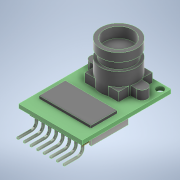
# Autodesk Inventor part: Camera
Saved by Autodesk Inventor 2022 (Build 260153000, 153)
## iProperties
Created: 2022-12-31
Part Number: Camera
Material: Generic
Document SubType Name: Modeling
Designer: karpova
Density: 1 g/cm^3
Appearance: Smooth - Dark Forest Green
Author: karpova
Autodesk Inventor part; units mm, degrees
ref_plane "YZ Plane" through (0, 0, 0) normal (1, 0, 0) x (0, 1, 0)
ref_plane "XZ Plane" through (0, 0, 0) normal (0, 1, 0) x (-1, 0, 0)
ref_plane "XY Plane" through (0, 0, 0) normal (0, 0, 1) x (1, 0, 0)
sketch "Sketch1" plane through (0, 0, 0) normal (0, 1, 0) x (-1, 0, 0)
  line L0 (0, 0) -> (34.25, 0)
  line L1 (34.25, 0) -> (34.25, -24.4)
  line L2 (34.25, -24.4) -> (0, -24.4)
  line L3 (0, -24.4) -> (0, 0)
  dimension "d0" = 24.4
  dimension "d1" = 34.25
  constraints: 8 end point, 2 parallel, 1 horizontal, 1 perpendicular
  measures "d0" distance of L0.end L1.end
  measures "d1" distance of L0.start L0.end
extrude "Extrusion1" add sketch "Sketch1" along normal blind 1.54
sketch "Sketch4" plane through (0, 1.54, 0) normal (0, 1, 0) x (1, 0, 0)
  line L0 (-32.8, 5.675) -> (-19.75, 5.675)
  line L1 (-19.75, 5.675) -> (-19.75, 18.725)
  line L2 (-19.75, 18.725) -> (-32.8, 18.725)
  line L3 (-32.8, 18.725) -> (-32.8, 5.675)
  circle A0 centre (-32.12, 2.2) radius 1.5 projected
  line L4 (-34.25, 24.4) -> (-34.25, 0) construction
  line L5 (-34.25, 12.2) -> (0, 12.2) construction
  line L6 (0, 0) -> (0, 24.4) construction
  line L7 (-26.275, 18.725) -> (-26.275, 5.675) construction
  line L8 (-28.325, 18.725) -> (-24.225, 18.725)
  line L9 (-24.225, 18.725) -> (-24.225, 21.2)
  line L10 (-26.275, 23.25) -> (-26.275, 23.25)
  line L11 (-28.325, 21.2) -> (-28.325, 18.725)
  line L12 (-24.225, 5.675) -> (-24.225, 3.2)
  line L13 (-26.275, 1.15) -> (-26.275, 1.15)
  line L14 (-28.325, 3.2) -> (-28.325, 5.675)
  arc A1 (-26.275, 23.25) -> (-28.325, 21.2) centre (-26.275, 21.2) ccw
  arc A2 (-24.225, 21.2) -> (-26.275, 23.25) centre (-26.275, 21.2) ccw
  arc A3 (-28.325, 3.2) -> (-26.275, 1.15) centre (-26.275, 3.2) ccw
  arc A4 (-26.275, 1.15) -> (-24.225, 3.2) centre (-26.275, 3.2) ccw
  point P0 (-24.225, 23.25)
  point P1 (-28.325, 23.25)
  point P2 (-24.225, 1.15)
  point P3 (-28.325, 1.15)
  point P4 (-26.275, 1.15)
  dimension "d43" = 13.05
  dimension "d44" = 14.5
  dimension "d56" = 4.1
  dimension "d57" = 22.1
  dimension "d58" = 2.05
  constraints: 26 end point, 9 point on line, 8 point on circle, 8 tangent, 4 centre point, 4 midpoint, 4 symmetric about line, 3 equal radius, 3 parallel, 3 perpendicular, 2 horizontal, 1 vertical, 2 other
  measures "d43" distance between parallel lines of L2 L0
  measures "d44" distance between parallel lines of L4 L1
  measures "d56" distance between parallel lines of L9 L11
  measures "d57" distance between parallel lines of L10 L13
  measures "d58" radius of A1
extrude "Extrusion2" add sketch "Sketch4" along normal blind 3.46 contours L3 L2 L1 L0 | L0 L12 A4 A3 L14 | L11 A1 A2 L9 L2
sketch "Sketch8" plane through (0, 1.54, 0) normal (0, 1, 0) x (1, 0, 0)
  line L0 (0, 24.4) -> (-34.25, 24.4) projected
  line L1 (0, 0) -> (0, 24.4) projected
  line L2 (-34.25, 0) -> (0, 0) projected
  line L3 (-34.25, 24.4) -> (-34.25, 0) projected
  line L4 (-32.8, 5.675) -> (-32.8, 18.725) construction
  line L5 (-32.8, 12.2) -> (-26.275, 12.2) construction
  line L6 (-26.275, 12.2) -> (-26.275, 18.725) construction
  line L7 (-32.8, 18.725) -> (-19.75, 18.725) construction
  circle A0 centre (-26.275, 12.2) radius 7
  dimension "d45" = 14
  constraints: 4 end point, 2 midpoint, 1 centre point, 1 coincident, 1 horizontal, 1 vertical
  measures "d45" diameter of A0
extrude "Extrusion6" add sketch "Sketch8" along normal blind 8.61 contours A0
sketch "Sketch9" plane through (-26.275, 10.15, -12.2) normal (0, 1, 0) x (1, 0, 0)
  circle A0 centre (0, 0) radius 7 projected
  circle A1 centre (0, 0) radius 5.875
  point P0 (26.275, -12.2)
  dimension "d48" = 11.75
  constraints: 1 centre point, 1 coincident
  measures "d48" diameter of A1
extrude "Extrusion7" add sketch "Sketch9" along normal blind 3.15 contours A1
sketch "Sketch10" plane through (-26.275, 13.3, -12.2) normal (0, 1, 0) x (1, 0, 0)
  circle A0 centre (0, 0) radius 5.875 projected
  circle A1 centre (0, 0) radius 7 projected
  point P0 (26.275, -12.2)
extrude "Extrusion8" add sketch "Sketch10" along normal blind 3.2 contours A0 | A1
sketch "Sketch11" plane through (-26.275, 16.5, -12.2) normal (0, 1, 0) x (1, 0, 0)
  circle A0 centre (0, 0) radius 7 projected
  circle A1 centre (0, 0) radius 5.45
  point P0 (26.275, -12.2)
  dimension "d53" = 10.9
  constraints: 1 centre point, 1 coincident
  measures "d53" diameter of A1
extrude "Extrusion9" cut sketch "Sketch11" against normal blind 4 contours A1
sketch "Sketch12" plane through (0, 1.54, 0) normal (0, 1, 0) x (1, 0, 0)
  circle A0 centre (-32.15, 2.1) radius 1.45
  line L0 (-34.25, 24.4) -> (-34.25, 0) construction
  line L1 (-34.25, 12.2) -> (0, 12.2) construction
  line L2 (0, 0) -> (0, 24.4) construction
  circle A1 centre (-32.15, 22.3) radius 1.45
  line L3 (-34.25, 0) -> (0, 0) projected
  dimension "d59" = 2.9
  dimension "d60" = 0.65
  dimension "d61" = 0.65
  constraints: 2 centre point, 2 end point, 2 midpoint, 1 symmetric about line, 1 other
  measures "d59" diameter of A0
  measures "d60" distance edge to line of A0 L0
  measures "d61" distance edge to line of A0 L3
extrude "Extrusion10" cut sketch "Sketch12" against normal through all
sketch "Sketch13" plane through (0, 1.54, 0) normal (0, 1, 0) x (1, 0, 0)
  line L0 (-15.7, 2.2219) -> (-5.6, 2.2219)
  line L1 (-5.6, 2.2219) -> (-5.6, 22.1781)
  line L2 (-5.6, 22.1781) -> (-15.7, 22.1781)
  line L3 (-15.7, 22.1781) -> (-15.7, 2.2219)
  line L4 (0, 0) -> (0, 24.4) construction
  line L5 (0, 12.2) -> (-34.25, 12.2) construction
  line L6 (-34.25, 24.4) -> (-34.25, 0) construction
  dimension "d64" = 15.7
  dimension "d65" = 10.1
  constraints: 10 end point, 2 midpoint, 2 parallel, 1 horizontal, 1 perpendicular, 1 other
  measures "d64" distance between parallel lines of L4 L3
  measures "d65" distance of L0.start L0.end
extrude "Extrusion11" add sketch "Sketch13" along normal blind 1.06
sketch "Sketch14" plane through (0, 0, 0) normal (0, -1, 0) x (1, 0, 0)
  line L0 (-8.6295, -19.3) -> (-22.8295, -19.3)
  line L1 (-22.8295, -19.3) -> (-22.8295, -4.9)
  line L2 (-22.8295, -4.9) -> (-8.6295, -4.9)
  line L3 (-8.6295, -4.9) -> (-8.6295, -19.3)
  line L4 (0, -24.4) -> (-34.25, -24.4) projected
  point P0 (0, 0)
  dimension "d68" = 14.2
  dimension "d69" = 14.4
  dimension "d70" = 19.5
  constraints: 8 end point, 2 parallel, 1 horizontal, 1 perpendicular
  measures "d68" distance of L0.start L0.end
  measures "d69" distance of L2.end L0.start
  measures "d70" distance between parallel lines of L4 L2
extrude "Extrusion12" add sketch "Sketch14" along normal blind 7.26
sketch "Sketch15" plane through (-8.6295, 0, -4.9) normal (1, 0, 0) x (0, 0, -1)
  line L0 (0, -7.26) -> (14.4, -7.26) projected
  line L1 (0.8, -7.26) -> (2.2, -7.26)
  line L2 (2.2, -7.26) -> (2.2, -3.31)
  line L3 (2.2, -3.31) -> (0.8, -3.31)
  line L4 (0.8, -3.31) -> (0.8, -7.26)
  line L5 (0, 0) -> (0, -7.26) projected
  line L6 (3.075, -7.26) -> (4.475, -7.26)
  line L7 (4.475, -7.26) -> (4.475, -3.31)
  line L8 (4.475, -3.31) -> (3.075, -3.31)
  line L9 (3.075, -3.31) -> (3.075, -7.26)
  line L10 (5.35, -7.26) -> (6.75, -7.26)
  line L11 (6.75, -7.26) -> (6.75, -3.31)
  line L12 (6.75, -3.31) -> (5.35, -3.31)
  line L13 (5.35, -3.31) -> (5.35, -7.26)
  line L14 (7.625, -7.26) -> (9.025, -7.26)
  line L15 (9.025, -7.26) -> (9.025, -3.31)
  line L16 (9.025, -3.31) -> (7.625, -3.31)
  line L17 (7.625, -3.31) -> (7.625, -7.26)
  line L18 (9.9, -7.26) -> (11.3, -7.26)
  line L19 (11.3, -7.26) -> (11.3, -3.31)
  line L20 (11.3, -3.31) -> (9.9, -3.31)
  line L21 (9.9, -3.31) -> (9.9, -7.26)
  line L22 (12.175, -7.26) -> (13.575, -7.26)
  line L23 (13.575, -7.26) -> (13.575, -3.31)
  line L24 (13.575, -3.31) -> (12.175, -3.31)
  line L25 (12.175, -3.31) -> (12.175, -7.26)
  point P0 (-4.9, 0)
  point P1 (2.2, -7.26)
  point P2 (3.075, -7.26)
  point P3 (5.35, -7.26)
  point P4 (6.75, -7.26)
  point P5 (7.625, -7.26)
  point P6 (9.025, -7.26)
  point P7 (12.175, -7.26)
  dimension "d73" = 3.95
  dimension "d74" = 0.8
  dimension "d75" = 1.4
  dimension "d78" = 2.275
  constraints: 48 end point, 2 horizontal, 2 parallel, 1 perpendicular, 1 point on line, 40 other
  measures "d73" distance between parallel lines of L0 L3
  measures "d74" distance between parallel lines of L5 L4
  measures "d75" distance between parallel lines of L4 L2
  measures "d78" distance of L1.start L6.start
extrude "Extrusion13" cut sketch "Sketch15" against normal through all
sketch "Sketch16" plane through (0, 0, 0) normal (0, -1, 0) x (1, 0, 0)
  line L0 (-2.2969, -2) -> (-4.7969, -2)
  line L1 (-4.7969, -2) -> (-4.7969, -22.3)
  line L2 (-4.7969, -22.3) -> (-2.2969, -22.3)
  line L3 (-2.2969, -22.3) -> (-2.2969, -2)
  line L4 (0, -24.4) -> (-34.25, -24.4) projected
  point P0 (0, 0)
  dimension "d85" = 20.3
  dimension "d86" = 2.5
  dimension "d87" = 22.4
  constraints: 8 end point, 2 parallel, 1 horizontal, 1 perpendicular
  measures "d85" distance of L2.end L0.start
  measures "d86" distance of L0.start L0.end
  measures "d87" distance between parallel lines of L4 L0
extrude "Extrusion14" add sketch "Sketch16" along normal blind 2.51
sketch "Sketch17" plane through (0, -2.51, 0) normal (0, -1, 0) x (1, 0, 0)
  line L0 (-3.2219, -21.3563) -> (-3.8719, -21.3563)
  line L1 (-3.8719, -21.3563) -> (-3.8719, -20.7063)
  line L2 (-3.8719, -20.7063) -> (-3.2219, -20.7063)
  line L3 (-3.2219, -20.7063) -> (-3.2219, -21.3563)
  line L4 (-2.2969, -22.3) -> (-4.7969, -22.3) construction
  line L5 (-3.5469, -22.3) -> (-3.5469, -2) construction
  line L6 (-4.7969, -2) -> (-2.2969, -2) construction
  line L7 (-2.2969, -2) -> (-2.2969, -22.3) construction
  line L8 (-2.2969, -19.7625) -> (-4.7969, -19.7625) construction
  line L9 (-4.7969, -22.3) -> (-4.7969, -2) construction
  line L10 (-2.2969, -21.0313) -> (-4.7969, -21.0313) construction
  line L11 (-3.2219, -18.8188) -> (-3.8719, -18.8188)
  line L12 (-3.8719, -18.8188) -> (-3.8719, -18.1688)
  line L13 (-3.8719, -18.1688) -> (-3.2219, -18.1688)
  line L14 (-3.2219, -18.1688) -> (-3.2219, -18.8188)
  line L15 (-3.2219, -16.2813) -> (-3.8719, -16.2813)
  line L16 (-3.8719, -16.2813) -> (-3.8719, -15.6313)
  line L17 (-3.8719, -15.6313) -> (-3.2219, -15.6313)
  line L18 (-3.2219, -15.6313) -> (-3.2219, -16.2813)
  line L19 (-3.2219, -13.7438) -> (-3.8719, -13.7438)
  line L20 (-3.8719, -13.7438) -> (-3.8719, -13.0938)
  line L21 (-3.8719, -13.0938) -> (-3.2219, -13.0938)
  line L22 (-3.2219, -13.0938) -> (-3.2219, -13.7438)
  line L23 (-3.2219, -11.2063) -> (-3.8719, -11.2063)
  line L24 (-3.8719, -11.2063) -> (-3.8719, -10.5563)
  line L25 (-3.8719, -10.5563) -> (-3.2219, -10.5563)
  line L26 (-3.2219, -10.5563) -> (-3.2219, -11.2063)
  line L27 (-3.2219, -8.6688) -> (-3.8719, -8.6688)
  line L28 (-3.8719, -8.6688) -> (-3.8719, -8.0188)
  line L29 (-3.8719, -8.0188) -> (-3.2219, -8.0188)
  line L30 (-3.2219, -8.0188) -> (-3.2219, -8.6688)
  line L31 (-3.2219, -6.1313) -> (-3.8719, -6.1313)
  line L32 (-3.8719, -6.1313) -> (-3.8719, -5.4813)
  line L33 (-3.8719, -5.4813) -> (-3.2219, -5.4813)
  line L34 (-3.2219, -5.4813) -> (-3.2219, -6.1313)
  line L35 (-3.2219, -3.5938) -> (-3.8719, -3.5938)
  line L36 (-3.8719, -3.5938) -> (-3.8719, -2.9438)
  line L37 (-3.8719, -2.9438) -> (-3.2219, -2.9438)
  line L38 (-3.2219, -2.9438) -> (-3.2219, -3.5938)
  point P0 (0, 0)
  dimension "d90" = 0.65
  dimension "d91" = 20.3
  dimension "d92" = 2.5375
  dimension "d95" = 2.5375
  constraints: 70 end point, 4 point on line, 3 horizontal, 2 midpoint, 2 parallel, 2 perpendicular, 1 vertical, 59 other
  measures "d90" distance of L0.start L0.end
  measures "d91" distance of L4.end L6.start
  measures "d92" distance between parallel lines of L4 L8
  measures "d95" distance of L0.start L11.start
ref_plane "Work Plane1" through (-2.2969, 0, -22.3) normal (0, 0, -1) x (-1, 0, 0)
sketch "Sketch18" plane through (-2.2969, 0, -22.3) normal (0, 0, -1) x (-1, 0, 0)
  line L0 (2.5, -2.51) -> (0, -2.51) projected
  line L1 (1.25, -2.51) -> (1.25, -4.5025)
  line L2 (-0.7425, -6.495) -> (-6.075, -6.495)
  arc A0 (-0.7425, -6.495) -> (1.25, -4.5025) centre (-0.7425, -4.5025) ccw
  point P0 (-2.2969, 0)
  point P1 (1.25, -6.495)
  dimension "d101" = 3.985
  dimension "d102" = 7.325
  dimension "d103" = 1.9925
  constraints: 4 end point, 2 point on circle, 2 point on line, 2 tangent, 1 centre point, 1 midpoint, 1 perpendicular, 1 vertical
  measures "d101" distance between parallel lines of L0 L2
  measures "d102" distance of point (1.25, -6.495) L2.end
  measures "d103" radius of A0
sweep "Sweep1" add profiles "Sketch17" path "Sketch18" path curves L1 A0 L2
equation "\"d2\" = pcbThickness"
equation "\"d58\" = 0.5 * d56"
equation "\"d92\" = 0.125 * d91"
equation "\"d95\" = 0.125 * d91"
equation "\"d103\" = 0.5 * d101"
equation "\"pcbThickness\" = 1.54"
body "Solid1"
